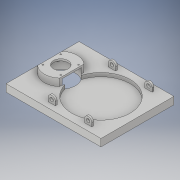
# Autodesk Inventor part: base
Saved by Autodesk Inventor 2019 (Build 230136000, 136)
## iProperties
Created: 2019-05-13
Part Number: base
Material: Generic
Document SubType Name: Modeling
Designer: Nathan
Density: 1 g/cm^3
Appearance: Default
Author: Nathan
Autodesk Inventor part; units mm, degrees
ref_plane "YZ Plane" through (0, 0, 0) normal (1, 0, 0) x (0, 1, 0)
ref_plane "XZ Plane" through (0, 0, 0) normal (0, 1, 0) x (-1, 0, 0)
ref_plane "XY Plane" through (0, 0, 0) normal (0, 0, 1) x (1, 0, 0)
sketch "Sketch1" plane through (0, 0, 0) normal (0, 1, 0) x (-1, 0, 0)
  line L0 (82.55, 63.5) -> (-82.55, 63.5)
  line L1 (-82.55, 63.5) -> (-82.55, -63.5)
  line L2 (-82.55, -63.5) -> (82.55, -63.5)
  line L3 (82.55, -63.5) -> (82.55, 63.5)
  line L4 (82.55, 63.5) -> (-82.55, -63.5) construction
  line L5 (-82.55, 63.5) -> (82.55, -63.5) construction
  point P0 (0, 0)
  dimension "d0" = 165.1
  dimension "d1" = 127
  constraints: 12 end point, 2 midpoint, 2 parallel, 1 horizontal, 1 perpendicular
  measures "d0" distance of L2.end L1.end
  measures "d1" distance of L1.end L0.end
extrude "Extrusion1" add sketch "Sketch1" along normal blind 12.7
sketch "Sketch2" plane through (0, 12.7, 0) normal (0, 1, 0) x (1, 0, 0)
  circle A0 centre (19.05, 0) radius 50.8
  line L0 (82.55, 63.5) -> (-82.55, 63.5) projected
  line L1 (82.55, -63.5) -> (82.55, 63.5) projected
  point P0 (0, 0)
  dimension "d4" = 101.6
  dimension "d5" = 63.5
  dimension "d6" = 63.5
  constraints: 1 centre point, 1 horizontal alignment
  measures "d4" diameter of A0
  measures "d5" distance from line of A0.centre L0
  measures "d6" distance from line of L1 A0.centre
extrude "Extrusion2" cut sketch "Sketch2" against normal blind 6.35
sketch "Sketch11" plane through (0, 12.7, 0) normal (0, 1, 0) x (1, 0, 0)
  arc A0 (69.85, 0) -> (69.85, 0) centre (19.05, 0) ccw projected
  line L0 (-19.05, 53.975) -> (-6.35, 53.975)
  line L1 (-6.35, 53.975) -> (-6.35, 50.8)
  line L2 (-6.35, 50.8) -> (-19.05, 50.8)
  line L3 (-19.05, 50.8) -> (-19.05, 53.975)
  line L4 (19.05, 0) -> (19.05, 50.8) construction
  line L5 (82.55, 63.5) -> (-82.55, 63.5) construction
  line L6 (19.05, 0) -> (69.85, 0) construction
  point P0 (0, 0)
  dimension "d38" = 12.7
  dimension "d39" = 3.175
  dimension "d40" = 50.8
  dimension "d41" = 25.4
  constraints: 12 end point, 2 parallel, 2 perpendicular, 2 point on circle, 1 horizontal
  measures "d38" distance of L0.start L0.end
  measures "d39" distance of L2.end L0.start
  measures "d40" distance between parallel lines of L6 L2
  measures "d41" distance between parallel lines of L4 L1
extrude "Extrusion6" add sketch "Sketch11" along normal blind 6.35 contours L0 L1 L2 L3
sketch "Sketch12" plane through (-19.05, 12.7, -50.8) normal (0, 0, 1) x (1, 0, 0)
  line L0 (0, 6.35) -> (12.7, 6.35) projected
  circle A0 centre (6.35, 6.35) radius 6.35
  point P0 (19.05, -12.7)
  constraints: 1 horizontal alignment, 1 midpoint, 2 other
extrude "Extrusion7" add sketch "Sketch12" against normal blind 3.175
sketch "Sketch13" plane through (-19.05, 12.7, -50.8) normal (0, 0, 1) x (1, 0, 0)
  arc A0 (12.7, 6.35) -> (0, 6.35) centre (6.35, 6.35) ccw projected
  point P0 (19.05, -12.7)
  constraints: 1 coincident
hole "Hole2" at (-12.7, 19.05, -50.8) direction (0, 0, -1) diameter 6.35 end through all
sketch "Sketch14" plane through (0, 6.35, 0) normal (0, 1, 0) x (1, 0, 0)
  arc A0 (69.85, 0) -> (69.85, 0) centre (19.05, 0) ccw projected
  arc A1 (69.85, 0) -> (69.85, 0) centre (19.05, 0) ccw construction
  line L0 (19.05, 50.8) -> (19.05, -50.8) construction
  line L1 (-31.75, 0) -> (69.85, 0) construction
  line L2 (82.55, -63.5) -> (82.55, 63.5) construction
  point P0 (0, 0)
  constraints: 4 end point, 4 point on circle, 2 midpoint, 1 parallel, 1 perpendicular
ref_plane "Work Plane2" through (19.05, 6.35, -50.8) normal (-1, 0, 0) x (0, 0, 1)
ref_plane "Work Plane3" through (-31.75, 6.35, 0) normal (0, 0, 1) x (1, 0, 0)
mirror "Mirror1" about plane through (19.05, 6.35, -50.8) normal (-1, 0, 0) of "Extrusion6", "Extrusion7", "Hole2"
mirror "Mirror2" about plane through (-31.75, 6.35, 0) normal (0, 0, 1) of "Extrusion6", "Extrusion7", "Hole2", "Mirror1"
sketch "Sketch15" plane through (0, 12.7, 0) normal (0, 1, 0) x (1, 0, 0)
  line L0 (57.15, -53.975) -> (44.45, -53.975) projected
  line L1 (44.45, -53.975) -> (44.45, -50.8) projected
  line L2 (44.45, -50.8) -> (57.15, -50.8) projected
  line L3 (57.15, -50.8) -> (57.15, -53.975) projected
  line L4 (-6.35, -53.975) -> (-19.05, -53.975) projected
  line L5 (-19.05, -53.975) -> (-19.05, -50.8) projected
  line L6 (-19.05, -50.8) -> (-6.35, -50.8) projected
  line L7 (-6.35, -50.8) -> (-6.35, -53.975) projected
  line L8 (44.45, 53.975) -> (57.15, 53.975) projected
  line L9 (57.15, 53.975) -> (57.15, 50.8) projected
  line L10 (57.15, 50.8) -> (44.45, 50.8) projected
  line L11 (44.45, 50.8) -> (44.45, 53.975) projected
  line L12 (-6.35, 53.975) -> (-6.35, 50.8) projected
  line L13 (-6.35, 50.8) -> (-19.05, 50.8) projected
  line L14 (-19.05, 50.8) -> (-19.05, 53.975) projected
  line L15 (-19.05, 53.975) -> (-6.35, 53.975) projected
  circle A0 centre (19.05, 0) radius 50.8 projected
  line L16 (-82.55, -63.5) -> (82.55, -63.5) projected
  line L17 (82.55, -63.5) -> (82.55, 63.5) projected
  line L18 (82.55, 63.5) -> (-82.55, 63.5) projected
  line L19 (-82.55, 63.5) -> (-82.55, -63.5) projected
  circle A1 centre (-50.8, 0) radius 25.4
  point P0 (0, 0)
  point P1 (-31.75, 0)
  point P2 (-25.4, 0)
  dimension "d55" = 50.8
  dimension "d56" = 6.35
  constraints: 5 horizontal alignment, 3 other
  measures "d56" distance of point (-25.4, 0) point (-31.75, 0)
extrude "Extrusion8" cut sketch "Sketch15" against normal blind 25.4 contours A1 A0 | A0 A1 picked at (-29.4828, 0) picked at (-46.3538, -1.0252)
sketch "Sketch19" plane through (0, 12.7, 0) normal (0, 1, 0) x (1, 0, 0)
  arc A0 (-29.7295, 14.1844) -> (-29.7295, -14.1844) centre (-50.8, 0) ccw projected
  line L0 (-50.8, -25.4) -> (-50.8, 25.4) construction
  line L1 (-69.85, -21.2985) -> (-69.85, -16.8005)
  line L2 (-31.75, -21.2985) -> (-31.75, -16.8005)
  arc A1 (-31.75, 16.8005) -> (-69.85, 16.8005) centre (-50.8, 0) ccw
  arc A2 (-69.85, -16.8005) -> (-31.75, -16.8005) centre (-50.8, 0) ccw
  circle A3 centre (-50.8, 0) radius 25.4 construction
  line L3 (-76.2, 0) -> (-25.4, 0) construction
  arc A4 (-69.85, -21.2985) -> (-31.75, -21.2985) centre (-50.8, 0) ccw
  arc A5 (-31.75, 21.2985) -> (-69.85, 21.2985) centre (-50.8, 0) ccw
  line L4 (-69.85, -16.8005) -> (-69.85, 16.8005) construction
  line L5 (-31.75, -16.8005) -> (-31.75, 16.8005) construction
  line L6 (-69.85, 16.8005) -> (-69.85, 21.2985)
  line L7 (-31.75, 16.8005) -> (-31.75, 21.2985)
  point P0 (0, 0)
  dimension "d6" = 63.5
  dimension "d79" = 19.05
  dimension "d80" = 0
  dimension "d81" = 3.175
  constraints: 16 end point, 12 point on circle, 9 parallel, 4 centre point, 4 vertical, 2 midpoint, 2 point on line, 1 coincident, 1 horizontal, 3 other
  measures "d79" distance between parallel lines of L0 L1
  measures "d80" radial gap between concentric circles of A1 A0
  measures "d81" radial gap between concentric circles of A4 A2
extrude "Extrusion12" add sketch "Sketch19" along normal blind 12.7
sketch "Sketch20" plane through (0, 25.4, 0) normal (0, 1, 0) x (1, 0, 0)
  arc A0 (-31.75, 16.8005) -> (-69.85, 16.8005) centre (-50.8, 0) ccw projected
  arc A1 (-69.85, -16.8005) -> (-31.75, -16.8005) centre (-50.8, 0) ccw projected
  line L0 (-69.85, -16.8005) -> (-69.85, 16.8005)
  line L1 (-31.75, -21.2985) -> (-31.75, -16.8005) projected
  line L2 (-31.75, 16.8005) -> (-31.75, -16.8005)
  arc A2 (-31.75, 16.8005) -> (-69.85, 16.8005) centre (-50.8, 0) ccw projected
  arc A3 (-31.75, 16.8005) -> (-69.85, 16.8005) centre (-50.8, 0) ccw
  arc A4 (-69.85, -16.8005) -> (-31.75, -16.8005) centre (-50.8, 0) ccw
  point P0 (0, 0)
  constraints: 4 end point, 4 point on circle, 2 centre point, 2 coincident, 2 vertical, 1 other
extrude "Extrusion13" add sketch "Sketch20" against normal blind 3.175
sketch "Sketch21" plane through (0, 25.4, 0) normal (0, 1, 0) x (1, 0, 0)
  arc A0 (-29.7295, 14.1844) -> (-29.7295, -14.1844) centre (-50.8, 0) ccw projected
  line L0 (-66.3, 15.5) -> (-35.3, 15.5) construction
  line L1 (-35.3, 15.5) -> (-35.3, -15.5) construction
  line L2 (-35.3, -15.5) -> (-66.3, -15.5) construction
  line L3 (-66.3, -15.5) -> (-66.3, 15.5) construction
  circle A1 centre (-50.8, 0) radius 12.7
  point P0 (0, 0)
  point P1 (-35.3, 0)
  point P2 (-50.8, 15.5)
  dimension "d86" = 31
  dimension "d87" = 31
  dimension "d95" = 25.4
  constraints: 8 end point, 5 coincident, 2 midpoint, 2 parallel, 1 centre point, 1 horizontal, 1 horizontal alignment, 1 perpendicular, 1 vertical alignment
  measures "d86" distance of L1.end L2.end
  measures "d87" distance of L0.end L1.end
  measures "d95" diameter of A1
hole "Hole4" at (-66.3, 25.4, -15.5) at (-35.3, 25.4, -15.5) at (-66.3, 25.4, 15.5) at (-35.3, 25.4, 15.5) direction (0, -1, 0) diameter 2.5 end through all
extrude "Extrusion14" cut sketch "Sketch21" against normal through all
equation "\"d0\" = base_width"
equation "\"d1\" = base_length"
equation "\"d2\" = base_height"
equation "\"d4\" = turntable_diameter"
equation "\"d6\" = d5"
equation "\"d7\" = turntable_bed_depth"
equation "\"d42\" = turntable_thickness - turntable_bed_depth + 0.5 * retention_poles_diameter"
equation "\"d46\" = retention_poles_diameter"
equation "\"d55\" = waist_motor_cutout_diameter"
equation "\"d56\" = waist_cutout_overlap"
equation "\"d81\" = base_motor_standoff_thickness"
equation "\"d82\" = base_motor_standoff_height"
equation "\"d84\" = base_motor_standoff_thickness"
equation "\"d96\" = base_motor_standoff_thickness"
equation "\"turntable_diameter\" = 101.6"
equation "\"turntable_spur_thickness\" = 6.35"
equation "\"turntable_thickness\" = 9.525"
equation "\"spine_diameter\" = 38.1"
equation "\"shoulder_height_offset\" = 25.4"
equation "\"shoulder_width\" = 63.5"
equation "\"shoulder_length\" = 50.8"
equation "\"shoulder_wall_thickness\" = 6.35"
equation "\"arm_proximal_gear_diameter\" = 63.5"
equation "\"arm_proximal_gear_thickness\" = 9.525"
equation "\"shoulder_motor_gear_diameter\" = 31.75"
equation "\"arm_proximal_length\" = 177.8"
equation "\"arm_proximal_width\" = 12.7"
equation "\"base_length\" = 127"
equation "\"base_width\" = 165.1"
equation "\"base_height\" = 12.7"
equation "\"retention_poles_diameter\" = 6.35"
equation "\"turntable_bed_depth\" = 6.35"
equation "\"waist_cutout_overlap\" = 6.35"
equation "\"waist_motor_cutout_diameter\" = 50.8"
equation "\"base_motor_standoff_thickness\" = 3.175"
equation "\"base_motor_standoff_length\" = 63.5"
equation "\"base_motor_standoff_height\" = 12.7"
equation "\"base_motor_standoff_offset\" = 0"
body "Solid1"
